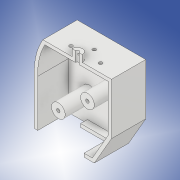
# Autodesk Inventor part: FA001
Saved by Autodesk Inventor 2017 SP1 (Build 210196100, 196)
## iProperties
Created: 2017-06-14
Part Number: FA001
Material: ABS Plastic
Document SubType Name: Modeling
Designer: zallen
Density: 1.06 g/cm^3
Appearance: CR White
Author: zallen
Autodesk Inventor part; units mm, degrees
ref_plane "YZ Plane" through (0, 0, 0) normal (1, 0, 0) x (0, 1, 0)
ref_plane "XZ Plane" through (0, 0, 0) normal (0, 1, 0) x (-1, 0, 0)
ref_plane "XY Plane" through (0, 0, 0) normal (0, 0, 1) x (1, 0, 0)
sketch "Sketch1" plane through (0, 0, 0) normal (0, 0, 1) x (1, 0, 0)
  line L0 (0, 0) -> (100, 0)
  line L1 (100, 0) -> (100, -75)
  line L2 (100, -75) -> (75, -118.3013)
  line L3 (-12.5, -50) -> (-12.5, -118.3013)
  arc A0 (0, 0) -> (-12.5, -50) centre (77.4072, -45.9143) ccw
  line L4 (-12.5, -118.3013) -> (75, -118.3013)
  dimension "d0" = 100
  dimension "d1" = 75
  dimension "d2" = 50
  dimension "d3" = 150
  dimension "d4" = 12.5
  dimension "d5" = 50
  dimension "d6" = 90
  constraints: 10 end point, 2 horizontal, 2 point on circle, 1 centre point, 1 horizontal alignment, 1 perpendicular, 1 vertical
  measures "d0" distance of L0.start L0.end
  measures "d1" distance of L0.end L1.end
  measures "d2" distance of L1.end L2.end
  measures "d3" angle of L1 L2
  measures "d4" horizontal distance of L0.start L3.start
  measures "d5" vertical distance of L0.start L3.start
  measures "d6" radius of A0
extrude "Extrusion1" add sketch "Sketch1" along normal blind 50
sketch "Sketch2" plane through (0, 0, 50) normal (0, 0, 1) x (1, 0, 0)
  line L0 (100, 0) -> (0, 0) projected
  arc A0 (0, 0) -> (-12.5, -50) centre (77.4072, -45.9143) ccw projected
  line L1 (-12.5, -50) -> (-12.5, -118.3013) projected
  line L2 (-12.5, -118.3013) -> (75, -118.3013) projected
  line L3 (75, -118.3013) -> (100, -75) projected
  line L4 (100, -75) -> (100, 0) projected
  arc A1 (2.902, -5) -> (-7.5, -49.8848) centre (77.4072, -45.9143) ccw
  line L5 (2.902, -5) -> (95, -5)
  line L6 (95, -5) -> (95, -73.6603)
  line L7 (95, -73.6603) -> (72.1132, -113.3013)
  line L8 (72.1132, -113.3013) -> (-7.5, -113.3013)
  line L9 (-7.5, -113.3013) -> (-7.5, -49.8848)
  dimension "d9" = 5
  constraints: 10 end point, 2 point on circle, 1 centre point, 5 other
  measures "d9" radial gap between concentric circles of A0 A1
extrude "Extrusion2" cut sketch "Sketch2" against normal blind 45 contours L5 L6 L7 L8 L9 A1
sketch "Sketch3" plane through (0, 0, 50) normal (0, 0, 1) x (1, 0, 0)
  line L0 (72.1132, -113.3013) -> (-7.5, -113.3013) projected
  line L1 (-12.5, -118.3013) -> (75, -118.3013) projected
  line L2 (-7.5, -113.3013) -> (60, -113.3013)
  line L3 (60, -113.3013) -> (60, -118.3013)
  line L4 (60, -118.3013) -> (-7.5, -118.3013)
  line L5 (-7.5, -118.3013) -> (-7.5, -113.3013)
  point P0 (0, 0)
  dimension "d13" = 15
  constraints: 8 end point, 2 parallel, 1 horizontal, 1 perpendicular, 1 point on line
  measures "d13" distance from line of L1.end L3
extrude "Extrusion3" cut sketch "Sketch3" against normal blind 45
sketch "Sketch4" plane through (0, 0, 0) normal (0, 1, 0) x (1, 0, 0)
  circle A0 centre (50, -50) radius 2.75
  line L0 (100, -50) -> (0, -50) projected
  point P0 (0, 0)
  dimension "d16" = 5.5
  constraints: 1 centre point, 1 coincident, 1 midpoint
  measures "d16" diameter of A0
extrude "Extrusion4" cut sketch "Sketch4" against normal through all
sketch "Sketch5" plane through (0, 0, 0) normal (0, 1, 0) x (1, 0, 0)
  arc A0 (52.75, -50) -> (47.25, -50) centre (50, -50) ccw projected
  circle A1 centre (50, -50) radius 25 construction
  circle A2 centre (50, -25) radius 2.5
  circle A3 centre (28.3494, -37.5) radius 2.5
  circle A4 centre (28.3494, -62.5) radius 2.5
  circle A5 centre (50, -75) radius 2.5
  circle A6 centre (71.6506, -62.5) radius 2.5
  circle A7 centre (71.6506, -37.5) radius 2.5
  point P0 (0, 0)
  dimension "d20" = 50
  dimension "d21" = 5
  dimension "d24" = 360
  constraints: 6 centre point, 2 vertical alignment, 1 coincident, 15 other
  measures "d21" diameter of A2
extrude "Extrusion5" cut sketch "Sketch5" against normal blind 5 contours A2 | A3 | A7
sketch "Sketch12" plane through (0, 0, 0) normal (0, 1, 0) x (1, 0, 0)
  arc A0 (52.75, -50) -> (47.25, -50) centre (50, -50) ccw projected
  circle A1 centre (50, -50) radius 7.5 construction
  line L0 (52.75, -50) -> (95, -50) projected
  arc A2 (57.5, -50) -> (42.5, -50) centre (50, -50) ccw
  line L1 (2.902, -50) -> (47.25, -50) projected
  line L2 (42.5, -50) -> (47.25, -50)
  line L3 (52.75, -50) -> (57.5, -50)
  point P0 (0, 0)
  dimension "d53" = 15
  constraints: 4 end point, 4 point on circle, 2 centre point, 2 collinear, 2 concentric, 1 coincident, 1 point on line
  measures "d53" diameter of A1
extrude "Extrusion11" add sketch "Sketch12" along normal blind 10
sketch "Sketch13" plane through (0, 0, 0) normal (0, 0, 1) x (1, 0, 0)
  line L0 (42.5, 0) -> (57.5, 0) projected
  line L1 (42.5, 0) -> (42.5, 10) projected
  line L2 (57.5, 10) -> (42.5, 10) projected
  line L3 (57.5, 0) -> (57.5, 10) projected
  circle A0 centre (50, 5) radius 1.5
  point P0 (0, 0)
  point P1 (57.5, 5)
  point P2 (50, 10)
  dimension "d56" = 3
  constraints: 2 midpoint, 1 centre point, 1 horizontal alignment, 1 vertical alignment
  measures "d56" diameter of A0
extrude "Extrusion12" cut sketch "Sketch13" along normal through all contours A0
sketch "Sketch17" plane through (-12.5, -118.3013, 0) normal (0, -1, 0) x (1, 0, 0)
  line L0 (72.5, 5) -> (32.5, 5)
  line L1 (32.5, 5) -> (32.5, 15)
  line L2 (32.5, 15) -> (72.5, 15)
  line L3 (72.5, 15) -> (72.5, 5)
  point P0 (12.5, 0)
  dimension "d68" = 40
  dimension "d69" = 10
  constraints: 8 end point, 2 parallel, 1 horizontal, 1 perpendicular
  measures "d68" distance of L1.end L2.end
  measures "d69" distance of L0.end L1.end
extrude "Extrusion16" add sketch "Sketch17" against normal blind 5
sketch "Sketch18" plane through (0, 0, 5) normal (0, 0, 1) x (1, 0, 0)
  circle A0 centre (65, -45) radius 10
  circle A1 centre (65, -45) radius 2.5
  line L0 (100, 0) -> (57.5, 0) projected
  line L1 (100, -75) -> (100, 0) projected
  circle A2 centre (22.5, -78.3013) radius 10
  circle A3 centre (22.5, -78.3013) radius 2.5
  line L2 (-12.5, -50) -> (-12.5, -118.3013) projected
  line L3 (20, -118.3013) -> (60, -118.3013) projected
  point P0 (0, 0)
  dimension "d72" = 20
  dimension "d73" = 5
  dimension "d74" = 45
  dimension "d75" = 35
  dimension "d76" = 20
  dimension "d77" = 5
  dimension "d78" = 35
  dimension "d79" = 40
  constraints: 4 centre point, 2 coincident
  measures "d72" diameter of A0
  measures "d73" diameter of A1
  measures "d74" distance from line of L0 A0.centre
  measures "d75" distance from line of L1 A0.centre
  measures "d76" diameter of A2
  measures "d77" diameter of A3
  measures "d78" distance from line of L2 A2.centre
  measures "d79" distance from line of L3 A2.centre
extrude "Extrusion17" add sketch "Sketch18" along normal blind 45
body "Solid1"
